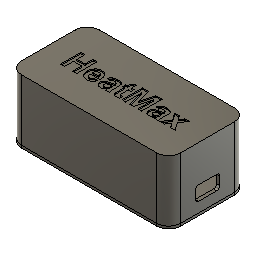
heatmax_box (Autodesk Fusion 360 design; units mm, degrees)
Autodesk Fusion 360 part; units mm, degrees
sketch "Sketch1" plane through (0, 0, 0) normal (0, 1, 0) x (1, 0, 0)
  line L0 (37.5, -17.5) -> (-37.5, -17.5)
  line L1 (-37.5, -17.5) -> (-37.5, 17.5)
  line L2 (-37.5, 17.5) -> (37.5, 17.5)
  line L3 (37.5, 17.5) -> (37.5, -17.5)
  line L4 (37.5, -17.5) -> (-37.5, 17.5) construction
  line L5 (-37.5, -17.5) -> (37.5, 17.5) construction
  line L6 (39.1, -19.1) -> (-39.1, -19.1)
  line L7 (-39.1, -19.1) -> (-39.1, 19.1)
  line L8 (-39.1, 19.1) -> (39.1, 19.1)
  line L9 (39.1, 19.1) -> (39.1, -19.1)
  dimension "d1" = 75
  dimension "d2" = 35
  dimension "d3" = -1.6
  constraint horizontal L0
  constraint perpendicular L0 L1
  constraint parallel L0 L2
  constraint parallel L1 L3
  constraint coincident L4 origin
  constraint coincident L5 origin
  measures "d1" distance of L1.end L2.end
  measures "d2" distance of L0.end L1.end
extrude "Extrude1" add sketch "Sketch1" along normal blind 30 makes body 1
sketch "Sketch2" plane through (0, 30, 0) normal (0, 1, 0) x (-1, 0, 0)
  line L0 (37.5, -17.5) -> (-37.5, -17.5)
  line L1 (-37.5, -17.5) -> (-37.5, 17.5)
  line L2 (-37.5, 17.5) -> (37.5, 17.5)
  line L3 (37.5, 17.5) -> (37.5, -17.5)
  line L4 (-39.1, -19.1) -> (39.1, -19.1)
  line L5 (39.1, -19.1) -> (39.1, 19.1)
  line L6 (39.1, 19.1) -> (-39.1, 19.1)
  line L7 (-39.1, 19.1) -> (-39.1, -19.1)
extrude "Extrude2" add sketch "Sketch2" against normal blind 1.6 contours L0 L1 L2 L3 bodies 1
fillet "Fillet1" radius 6 4 edges at (-39.1, 15, 19.1) (-39.1, 15, -19.1) (39.1, 15, -19.1) (39.1, 15, 19.1) on bodies 1
fillet "Fillet1" radius 5 4 edges at (37.5, 14.2, 17.5) (37.5, 14.2, -17.5) (-37.5, 14.2, -17.5) (-37.5, 14.2, 17.5) on bodies 1
sketch "Sketch3" plane through (0, 0, 0) normal (0, -1, 0) x (1, 0, 0)
  arc A0 (-37.5, -12.5) -> (-32.5, -17.5) centre (-32.5, -12.5) ccw
  line L0 (-37.5, -12.5) -> (-37.5, 12.5)
  arc A1 (-32.5, 17.5) -> (-37.5, 12.5) centre (-32.5, 12.5) ccw
  line L1 (-32.5, 17.5) -> (32.5, 17.5)
  arc A2 (37.5, 12.5) -> (32.5, 17.5) centre (32.5, 12.5) ccw
  line L2 (37.5, 12.5) -> (37.5, -12.5)
  arc A3 (32.5, -17.5) -> (37.5, -12.5) centre (32.5, -12.5) ccw
  line L3 (32.5, -17.5) -> (-32.5, -17.5)
  arc A4 (39.1, 13.1) -> (33.1, 19.1) centre (33.1, 13.1) ccw
  line L4 (33.1, 19.1) -> (-33.1, 19.1)
  arc A5 (-33.1, 19.1) -> (-39.1, 13.1) centre (-33.1, 13.1) ccw
  line L5 (-39.1, 13.1) -> (-39.1, -13.1)
  arc A6 (-39.1, -13.1) -> (-33.1, -19.1) centre (-33.1, -13.1) ccw
  line L6 (-33.1, -19.1) -> (33.1, -19.1)
  arc A7 (33.1, -19.1) -> (39.1, -13.1) centre (33.1, -13.1) ccw
  line L7 (39.1, -13.1) -> (39.1, 13.1)
  arc A8 (-37.4, -12.5) -> (-32.5, -17.4) centre (-32.5, -12.5) ccw
  line L8 (32.5, -17.4) -> (-32.5, -17.4)
  arc A9 (32.5, -17.4) -> (37.4, -12.5) centre (32.5, -12.5) ccw
  line L9 (37.4, 12.5) -> (37.4, -12.5)
  arc A10 (37.4, 12.5) -> (32.5, 17.4) centre (32.5, 12.5) ccw
  line L10 (-32.5, 17.4) -> (32.5, 17.4)
  arc A11 (-32.5, 17.4) -> (-37.4, 12.5) centre (-32.5, 12.5) ccw
  line L11 (-37.4, -12.5) -> (-37.4, 12.5)
  line L12 (37, 12.5) -> (37, -12.5)
  arc A12 (32.5, -17) -> (37, -12.5) centre (32.5, -12.5) ccw
  line L13 (32.5, -17) -> (-32.5, -17)
  arc A13 (-37, -12.5) -> (-32.5, -17) centre (-32.5, -12.5) ccw
  line L14 (-37, -12.5) -> (-37, 12.5)
  arc A14 (-32.5, 17) -> (-37, 12.5) centre (-32.5, 12.5) ccw
  line L15 (-32.5, 17) -> (32.5, 17)
  arc A15 (37, 12.5) -> (32.5, 17) centre (32.5, 12.5) ccw
  dimension "d12" = 0.1
  dimension "d13" = -0.5
extrude "Extrude3" add sketch "Sketch3" against normal blind 2 separate body contours A8 L8 A9 L9 A10 L10 A11 L11 makes body 2
sketch "Sketch4" plane through (0, 0, 0) normal (0, -1, 0) x (1, 0, 0)
  arc A0 (-37.5, -12.5) -> (-32.5, -17.5) centre (-32.5, -12.5) ccw
  line L0 (-37.5, -12.5) -> (-37.5, 12.5)
  arc A1 (-32.5, 17.5) -> (-37.5, 12.5) centre (-32.5, 12.5) ccw
  line L1 (-32.5, 17.5) -> (32.5, 17.5)
  arc A2 (37.5, 12.5) -> (32.5, 17.5) centre (32.5, 12.5) ccw
  line L2 (37.5, 12.5) -> (37.5, -12.5)
  arc A3 (32.5, -17.5) -> (37.5, -12.5) centre (32.5, -12.5) ccw
  line L3 (32.5, -17.5) -> (-32.5, -17.5)
  arc A4 (39.1, 13.1) -> (33.1, 19.1) centre (33.1, 13.1) ccw
  line L4 (33.1, 19.1) -> (-33.1, 19.1)
  arc A5 (-33.1, 19.1) -> (-39.1, 13.1) centre (-33.1, 13.1) ccw
  line L5 (-39.1, 13.1) -> (-39.1, -13.1)
  arc A6 (-39.1, -13.1) -> (-33.1, -19.1) centre (-33.1, -13.1) ccw
  line L6 (-33.1, -19.1) -> (33.1, -19.1)
  arc A7 (33.1, -19.1) -> (39.1, -13.1) centre (33.1, -13.1) ccw
  line L7 (39.1, -13.1) -> (39.1, 13.1)
extrude "Extrude4" add sketch "Sketch4" along normal blind 1.2 separate body contours A0 L0 A1 L1 A2 L2 A3 L3 | A4 L4 A5 L5 A6 L6 A7 L7 makes body 3
combine "Combine1" operation add target body 2 tool bodies 3
extrude "Extrude5" add 1 faces at (-10.8333, 2, -17.1333) along direction (0, 1, 0) blind 1 on bodies 2 bodies 2
sketch "Sketch5" plane through (39.1, 0, 0) normal (1, 0, 0) x (0, 0, -1)
  line L0 (-13.1, 30) -> (-13.1, 0)
  line L1 (-13.1, 0) -> (13.1, 0)
  line L2 (13.1, 0) -> (13.1, 30)
  line L3 (13.1, 30) -> (-13.1, 30)
  line L4 (0, 0) -> (0, 8.5) construction
  line L5 (6, 5) -> (-6, 5)
  line L6 (-6, 5) -> (-6, 12)
  line L7 (-6, 12) -> (6, 12)
  line L8 (6, 12) -> (6, 5)
  line L9 (6, 5) -> (-6, 12) construction
  line L10 (-6, 5) -> (6, 12) construction
  point P0 (0, 8.5)
  dimension "d20" = 12
  dimension "d21" = 7
  dimension "d22" = 5
  constraint coincident L4.start origin
  constraint perpendicular L1 L4
  constraint horizontal L5
  constraint perpendicular L5 L6
  constraint parallel L5 L7
  constraint parallel L6 L8
  constraint coincident L9 P0
  constraint coincident L10 P0
  constraint coincident P0 L4.end
  measures "d20" distance of L6.end L7.end
  measures "d21" distance of L5.end L6.end
  measures "d22" distance of L1 L5
extrude "Extrude6" cut sketch "Sketch5" against normal blind 3 contours L5 L6 L7 L8 bodies 1
fillet "Fillet2" radius 1.5 4 edges at (38.3, 12, 6) (38.3, 12, -6) (38.3, 5, -6) (38.3, 5, 6) on bodies 1
sketch "Sketch6" plane through (-39.1, 0, 0) normal (-1, 0, 0) x (0, 0, 1)
  line L0 (-13.1, 30) -> (-13.1, 0)
  line L1 (-13.1, 0) -> (13.1, 0)
  line L2 (13.1, 0) -> (13.1, 30)
  line L3 (13.1, 30) -> (-13.1, 30)
  line L4 (-4.5, 5) -> (4.5, 5)
  line L5 (0, 5) -> (0, 7) construction
  line L6 (5, 5) -> (-5, 5)
  line L7 (-5, 5) -> (-5, 9)
  line L8 (-5, 9) -> (5, 9)
  line L9 (5, 9) -> (5, 5)
  line L10 (5, 5) -> (-5, 9) construction
  line L11 (-5, 5) -> (5, 9) construction
  point P0 (0, 7)
  dimension "d27" = 4
  dimension "d28" = 10
  dimension "d29" = 2
  constraint midpoint L4 L5.start
  constraint perpendicular L4 L5
  constraint horizontal L6
  constraint perpendicular L6 L7
  constraint parallel L6 L8
  constraint parallel L7 L9
  constraint coincident L10 P0
  constraint coincident L11 P0
  constraint coincident P0 L5.end
  measures "d27" distance of L6.end L7.end
  measures "d28" distance of L7.end L8.end
  measures "d29" distance of L4 P0
extrude "Extrude7" cut sketch "Sketch6" against normal blind 3 contours L4 L6 L7 L8 L9 bodies 1
fillet "Fillet3" radius 1 4 edges at (-38.3, 9, 5) (-38.3, 9, -5) (-38.3, 5, -5) (-38.3, 5, 5) on bodies 1
sketch "Sketch7" plane through (0, 30, 0) normal (0, 1, 0) x (-1, 0, 0)
  arc A0 (-33.1, 19.1) -> (-39.1, 13.1) centre (-33.1, 13.1) ccw
  line L0 (-39.1, 13.1) -> (-39.1, -13.1)
  arc A1 (-39.1, -13.1) -> (-33.1, -19.1) centre (-33.1, -13.1) ccw
  line L1 (-33.1, -19.1) -> (33.1, -19.1)
  arc A2 (33.1, -19.1) -> (39.1, -13.1) centre (33.1, -13.1) ccw
  line L2 (39.1, -13.1) -> (39.1, 13.1)
  arc A3 (39.1, 13.1) -> (33.1, 19.1) centre (33.1, 13.1) ccw
  line L3 (33.1, 19.1) -> (-33.1, 19.1)
  line L4 (-35, 15) -> (35, 15)
  line L5 (35, 15) -> (35, -15)
  line L6 (35, -15) -> (-35, -15)
  line L7 (-35, -15) -> (-35, 15)
  line L8 (-35, 15) -> (35, -15) construction
  line L9 (35, 15) -> (-35, -15) construction
  line L10 (35, 15) -> (-35, 15) construction
  line L11 (-35, 15) -> (-35, -15) construction
  line L12 (-35, -15) -> (35, -15) construction
  line L13 (35, -15) -> (35, 15) construction
  dimension "d34" = 30
  dimension "d35" = 70
  dimension "d36" = 10
  text T0 "HeatMax" font "Arial" height 10 bold align centre middle in box 70 x 30 at (35, 15) x (-1, 0) y (0, -1) spacing 1
  constraint horizontal L4
  constraint perpendicular L4 L5
  constraint parallel L4 L6
  constraint parallel L5 L7
  constraint coincident L8 origin
  constraint coincident L9 origin
  constraint coincident L4.start
  constraint coincident L5.end
  measures "d34" distance of L4.end L5.end
  measures "d35" distance of L5.end L6.end
extrude "Extrude8" cut sketch "Sketch7" against normal blind 0.6 text T0 bodies 1
